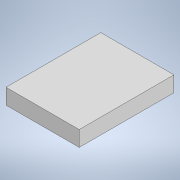
# Autodesk Inventor part: TPA2016
Saved by Autodesk Inventor 2022 (Build 260153000, 153)
## iProperties
Created: 2021-10-07
Part Number: TPA2016
Material: Generic
Document SubType Name: Modeling
Designer: ISS
Density: 1 g/cm^3
Appearance: Default
Author: ISS
Autodesk Inventor part; units mm, degrees
ref_plane "YZ Plane" through (0, 0, 0) normal (1, 0, 0) x (0, 1, 0)
ref_plane "XZ Plane" through (0, 0, 0) normal (0, 1, 0) x (-1, 0, 0)
ref_plane "XY Plane" through (0, 0, 0) normal (0, 0, 1) x (1, 0, 0)
sketch "Sketch1" plane through (0, 0, 0) normal (0, 1, 0) x (-1, 0, 0)
  line L0 (4.2156, 9.6325) -> (-17.3744, 9.6325)
  line L1 (-17.3744, 9.6325) -> (-17.3744, -18.3075)
  line L2 (-17.3744, -18.3075) -> (4.2156, -18.3075)
  line L3 (4.2156, -18.3075) -> (4.2156, 9.6325)
  point P0 (0, 0)
  dimension "d0" = 21.59
  dimension "d1" = 27.94
  constraints: 8 end point, 2 parallel, 1 horizontal, 1 perpendicular
  measures "d0" distance of L2.end L1.end
  measures "d1" distance of L1.end L0.end
extrude "Extrusion1" add sketch "Sketch1" along normal blind 4.572
body "Solid1"
